Autodesk Fusion 360 part; units mm, degrees
(part 2 of 2)
  arc A38 (5.901, -3.7653) -> (6.2114, -3.2278) centre (0, 0) ccw
  spline S19 degree 5 poles (5.2406, -2.0798) (5.2443, -2.0812) (5.2517, -2.0843) (5.2626, -2.0893) (5.2768, -2.0965) (5.2942, -2.1064) (5.3113, -2.117) (5.3283, -2.128) (5.3451, -2.1393) (5.3619, -2.1506) (5.3786, -2.1622) (5.3952, -2.174) (5.4117, -2.186) (5.428, -2.1983) (5.4442, -2.211) (5.4602, -2.2239) (5.4761, -2.2372) (5.4919, -2.2506) (5.5076, -2.2642) (5.5232, -2.278) (5.5387, -2.2919) (5.5541, -2.3061) (5.5694, -2.3204) (5.5846, -2.3349) (5.5997, -2.3497) (5.6147, -2.3646) (5.6296, -2.3797) (5.6444, -2.395) (5.6591, -2.4104) (5.6737, -2.426) (5.6882, -2.4418) (5.7026, -2.4577) (5.717, -2.4738) (5.7312, -2.49) (5.7453, -2.5064) (5.7593, -2.5229) (5.7733, -2.5396) (5.7871, -2.5565) (5.8008, -2.5735) (5.8145, -2.5906) (5.828, -2.6079) (5.8415, -2.6253) (5.8549, -2.6428) (5.8681, -2.6605) (5.8813, -2.6784) (5.8944, -2.6963) (5.9074, -2.7144) (5.9203, -2.7326) (5.9331, -2.751) (5.9458, -2.7695) (5.9584, -2.7881) (5.9709, -2.8068) (5.9833, -2.8257) (5.9956, -2.8447) (6.0078, -2.8638) (6.02, -2.8831) (6.032, -2.9024) (6.0439, -2.9219) (6.0558, -2.9415) (6.0675, -2.9612) (6.0792, -2.981) (6.0907, -3.001) (6.1022, -3.0211) (6.1135, -3.0412) (6.1248, -3.0615) (6.136, -3.0819) (6.147, -3.1024) (6.158, -3.123) (6.1689, -3.1438) (6.1797, -3.1646) (6.1903, -3.1856) (6.1988, -3.2024) (6.2051, -3.2151) (6.2093, -3.2235) (6.2114, -3.2278) knots 0 0 0 0 0 0 0.01428571 0.02857143 0.04285714 0.05714286 0.07142857 0.08571429 0.1 0.11428571 0.12857143 0.14285714 0.15714286 0.17142857 0.18571429 0.2 0.21428571 0.22857143 0.24285714 0.25714286 0.27142857 0.28571429 0.3 0.31428571 0.32857143 0.34285714 0.35714286 0.37142857 0.38571429 0.4 0.41428571 0.42857143 0.44285714 0.45714286 0.47142857 0.48571429 0.5 0.51428571 0.52857143 0.54285714 0.55714286 0.57142857 0.58571429 0.6 0.61428571 0.62857143 0.64285714 0.65714286 0.67142857 0.68571429 0.7 0.71428571 0.72857143 0.74285714 0.75714286 0.77142857 0.78571429 0.8 0.81428571 0.82857143 0.84285714 0.85714286 0.87142857 0.88571429 0.9 0.91428571 0.92857143 0.94285714 0.95714286 0.97142857 0.98571429 1 1 1 1 1 1
  line L19 (5.2406, -2.0798) -> (4.8563, -1.9265)
  arc A39 (4.5613, -1.3228) -> (4.8563, -1.9265) centre (5.0415, -1.4621) ccw
  arc A40 (4.5613, -1.3228) -> (4.6116, -1.135) centre (0, 0) ccw
  arc A41 (5.1689, -0.7597) -> (4.6116, -1.135) centre (5.0971, -1.2545) ccw
  line L20 (5.1689, -0.7597) -> (5.5783, -0.8192)
  spline S20 degree 5 poles (5.5783, -0.8192) (5.5823, -0.8197) (5.5902, -0.8208) (5.6021, -0.8219) (5.6181, -0.8228) (5.6381, -0.8229) (5.6583, -0.8223) (5.6784, -0.8212) (5.6986, -0.8199) (5.7188, -0.8184) (5.7391, -0.8168) (5.7593, -0.8149) (5.7796, -0.8127) (5.7999, -0.8102) (5.8203, -0.8073) (5.8406, -0.8041) (5.861, -0.8006) (5.8814, -0.7969) (5.9018, -0.793) (5.9222, -0.7888) (5.9426, -0.7845) (5.9631, -0.7799) (5.9835, -0.7752) (6.0039, -0.7702) (6.0244, -0.765) (6.0448, -0.7596) (6.0653, -0.7539) (6.0857, -0.7481) (6.1061, -0.7421) (6.1266, -0.7359) (6.147, -0.7295) (6.1675, -0.7229) (6.1879, -0.7161) (6.2083, -0.7092) (6.2288, -0.7021) (6.2492, -0.6947) (6.2696, -0.6873) (6.29, -0.6796) (6.3104, -0.6717) (6.3308, -0.6637) (6.3512, -0.6555) (6.3715, -0.6472) (6.3919, -0.6387) (6.4122, -0.63) (6.4325, -0.6211) (6.4528, -0.6121) (6.4731, -0.6029) (6.4934, -0.5936) (6.5137, -0.5841) (6.5339, -0.5744) (6.5541, -0.5646) (6.5743, -0.5546) (6.5945, -0.5445) (6.6147, -0.5342) (6.6348, -0.5238) (6.655, -0.5132) (6.6751, -0.5024) (6.6951, -0.4915) (6.7152, -0.4805) (6.7352, -0.4693) (6.7552, -0.4579) (6.7752, -0.4464) (6.7952, -0.4348) (6.8151, -0.423) (6.835, -0.4111) (6.8549, -0.399) (6.8747, -0.3867) (6.8945, -0.3744) (6.9143, -0.3619) (6.9341, -0.3492) (6.9538, -0.3364) (6.9695, -0.3261) (6.9813, -0.3182) (6.9892, -0.313) (6.9931, -0.3103) knots 0 0 0 0 0 0 0.01428571 0.02857143 0.04285714 0.05714286 0.07142857 0.08571429 0.1 0.11428571 0.12857143 0.14285714 0.15714286 0.17142857 0.18571429 0.2 0.21428571 0.22857143 0.24285714 0.25714286 0.27142857 0.28571429 0.3 0.31428571 0.32857143 0.34285714 0.35714286 0.37142857 0.38571429 0.4 0.41428571 0.42857143 0.44285714 0.45714286 0.47142857 0.48571429 0.5 0.51428571 0.52857143 0.54285714 0.55714286 0.57142857 0.58571429 0.6 0.61428571 0.62857143 0.64285714 0.65714286 0.67142857 0.68571429 0.7 0.71428571 0.72857143 0.74285714 0.75714286 0.77142857 0.78571429 0.8 0.81428571 0.82857143 0.84285714 0.85714286 0.87142857 0.88571429 0.9 0.91428571 0.92857143 0.94285714 0.95714286 0.97142857 0.98571429 1 1 1 1 1 1
  arc A42 (6.9931, -0.3103) -> (6.9931, 0.3103) centre (0, 0) ccw
  spline S21 degree 5 poles (5.5783, 0.8192) (5.5823, 0.8197) (5.5902, 0.8208) (5.6021, 0.8219) (5.6181, 0.8228) (5.6381, 0.8229) (5.6583, 0.8223) (5.6784, 0.8212) (5.6986, 0.8199) (5.7188, 0.8184) (5.7391, 0.8168) (5.7593, 0.8149) (5.7796, 0.8127) (5.7999, 0.8102) (5.8203, 0.8073) (5.8406, 0.8041) (5.861, 0.8006) (5.8814, 0.7969) (5.9018, 0.793) (5.9222, 0.7888) (5.9426, 0.7845) (5.9631, 0.7799) (5.9835, 0.7752) (6.0039, 0.7702) (6.0244, 0.765) (6.0448, 0.7596) (6.0653, 0.7539) (6.0857, 0.7481) (6.1061, 0.7421) (6.1266, 0.7359) (6.147, 0.7295) (6.1675, 0.7229) (6.1879, 0.7161) (6.2083, 0.7092) (6.2288, 0.7021) (6.2492, 0.6947) (6.2696, 0.6873) (6.29, 0.6796) (6.3104, 0.6717) (6.3308, 0.6637) (6.3512, 0.6555) (6.3715, 0.6472) (6.3919, 0.6387) (6.4122, 0.63) (6.4325, 0.6211) (6.4528, 0.6121) (6.4731, 0.6029) (6.4934, 0.5936) (6.5137, 0.5841) (6.5339, 0.5744) (6.5541, 0.5646) (6.5743, 0.5546) (6.5945, 0.5445) (6.6147, 0.5342) (6.6348, 0.5238) (6.655, 0.5132) (6.6751, 0.5024) (6.6951, 0.4915) (6.7152, 0.4805) (6.7352, 0.4693) (6.7552, 0.4579) (6.7752, 0.4464) (6.7952, 0.4348) (6.8151, 0.423) (6.835, 0.4111) (6.8549, 0.399) (6.8747, 0.3867) (6.8945, 0.3744) (6.9143, 0.3619) (6.9341, 0.3492) (6.9538, 0.3364) (6.9695, 0.3261) (6.9813, 0.3182) (6.9892, 0.313) (6.9931, 0.3103) knots 0 0 0 0 0 0 0.01428571 0.02857143 0.04285714 0.05714286 0.07142857 0.08571429 0.1 0.11428571 0.12857143 0.14285714 0.15714286 0.17142857 0.18571429 0.2 0.21428571 0.22857143 0.24285714 0.25714286 0.27142857 0.28571429 0.3 0.31428571 0.32857143 0.34285714 0.35714286 0.37142857 0.38571429 0.4 0.41428571 0.42857143 0.44285714 0.45714286 0.47142857 0.48571429 0.5 0.51428571 0.52857143 0.54285714 0.55714286 0.57142857 0.58571429 0.6 0.61428571 0.62857143 0.64285714 0.65714286 0.67142857 0.68571429 0.7 0.71428571 0.72857143 0.74285714 0.75714286 0.77142857 0.78571429 0.8 0.81428571 0.82857143 0.84285714 0.85714286 0.87142857 0.88571429 0.9 0.91428571 0.92857143 0.94285714 0.95714286 0.97142857 0.98571429 1 1 1 1 1 1
  line L21 (5.5783, 0.8192) -> (5.1689, 0.7597)
  arc A43 (4.6116, 1.135) -> (5.1689, 0.7597) centre (5.0971, 1.2545) ccw
  arc A44 (4.6116, 1.135) -> (4.5613, 1.3228) centre (0, 0) ccw
  arc A45 (4.8563, 1.9265) -> (4.5613, 1.3228) centre (5.0415, 1.4621) ccw
  line L22 (4.8563, 1.9265) -> (5.2406, 2.0798)
  spline S22 degree 5 poles (5.2406, 2.0798) (5.2443, 2.0812) (5.2517, 2.0843) (5.2626, 2.0893) (5.2768, 2.0965) (5.2942, 2.1064) (5.3113, 2.117) (5.3283, 2.128) (5.3451, 2.1393) (5.3619, 2.1506) (5.3786, 2.1622) (5.3952, 2.174) (5.4117, 2.186) (5.428, 2.1983) (5.4442, 2.211) (5.4602, 2.2239) (5.4761, 2.2372) (5.4919, 2.2506) (5.5076, 2.2642) (5.5232, 2.278) (5.5387, 2.2919) (5.5541, 2.3061) (5.5694, 2.3204) (5.5846, 2.3349) (5.5997, 2.3497) (5.6147, 2.3646) (5.6296, 2.3797) (5.6444, 2.395) (5.6591, 2.4104) (5.6737, 2.426) (5.6882, 2.4418) (5.7026, 2.4577) (5.717, 2.4738) (5.7312, 2.49) (5.7453, 2.5064) (5.7593, 2.5229) (5.7733, 2.5396) (5.7871, 2.5565) (5.8008, 2.5735) (5.8145, 2.5906) (5.828, 2.6079) (5.8415, 2.6253) (5.8549, 2.6428) (5.8681, 2.6605) (5.8813, 2.6784) (5.8944, 2.6963) (5.9074, 2.7144) (5.9203, 2.7326) (5.9331, 2.751) (5.9458, 2.7695) (5.9584, 2.7881) (5.9709, 2.8068) (5.9833, 2.8257) (5.9956, 2.8447) (6.0078, 2.8638) (6.02, 2.8831) (6.032, 2.9024) (6.0439, 2.9219) (6.0558, 2.9415) (6.0675, 2.9612) (6.0792, 2.981) (6.0907, 3.001) (6.1022, 3.0211) (6.1135, 3.0412) (6.1248, 3.0615) (6.136, 3.0819) (6.147, 3.1024) (6.158, 3.123) (6.1689, 3.1438) (6.1797, 3.1646) (6.1903, 3.1856) (6.1988, 3.2024) (6.2051, 3.2151) (6.2093, 3.2235) (6.2114, 3.2278) knots 0 0 0 0 0 0 0.01428571 0.02857143 0.04285714 0.05714286 0.07142857 0.08571429 0.1 0.11428571 0.12857143 0.14285714 0.15714286 0.17142857 0.18571429 0.2 0.21428571 0.22857143 0.24285714 0.25714286 0.27142857 0.28571429 0.3 0.31428571 0.32857143 0.34285714 0.35714286 0.37142857 0.38571429 0.4 0.41428571 0.42857143 0.44285714 0.45714286 0.47142857 0.48571429 0.5 0.51428571 0.52857143 0.54285714 0.55714286 0.57142857 0.58571429 0.6 0.61428571 0.62857143 0.64285714 0.65714286 0.67142857 0.68571429 0.7 0.71428571 0.72857143 0.74285714 0.75714286 0.77142857 0.78571429 0.8 0.81428571 0.82857143 0.84285714 0.85714286 0.87142857 0.88571429 0.9 0.91428571 0.92857143 0.94285714 0.95714286 0.97142857 0.98571429 1 1 1 1 1 1
  arc A46 (6.2114, 3.2278) -> (5.901, 3.7653) centre (0, 0) ccw
  spline S23 degree 5 poles (4.4214, 3.4986) (4.4245, 3.5011) (4.4309, 3.5059) (4.4406, 3.5129) (4.454, 3.5216) (4.4713, 3.5317) (4.4891, 3.5412) (4.5071, 3.5504) (4.5252, 3.5594) (4.5434, 3.5682) (4.5618, 3.5769) (4.5803, 3.5854) (4.599, 3.5936) (4.6178, 3.6016) (4.6369, 3.6093) (4.6561, 3.6167) (4.6755, 3.6239) (4.695, 3.6308) (4.7146, 3.6376) (4.7344, 3.6442) (4.7542, 3.6507) (4.7742, 3.657) (4.7943, 3.6631) (4.8144, 3.669) (4.8348, 3.6747) (4.8552, 3.6802) (4.8757, 3.6856) (4.8963, 3.6907) (4.917, 3.6957) (4.9378, 3.7006) (4.9587, 3.7053) (4.9797, 3.7098) (5.0008, 3.7142) (5.022, 3.7184) (5.0432, 3.7224) (5.0646, 3.7263) (5.086, 3.73) (5.1075, 3.7335) (5.1291, 3.7369) (5.1508, 3.7402) (5.1725, 3.7433) (5.1943, 3.7462) (5.2162, 3.749) (5.2381, 3.7517) (5.2602, 3.7542) (5.2823, 3.7565) (5.3044, 3.7587) (5.3267, 3.7608) (5.349, 3.7627) (5.3713, 3.7644) (5.3937, 3.766) (5.4162, 3.7675) (5.4388, 3.7688) (5.4614, 3.77) (5.4841, 3.771) (5.5068, 3.7719) (5.5296, 3.7726) (5.5524, 3.7732) (5.5753, 3.7737) (5.5982, 3.774) (5.6212, 3.7742) (5.6443, 3.7742) (5.6674, 3.7741) (5.6906, 3.7739) (5.7138, 3.7735) (5.737, 3.773) (5.7603, 3.7723) (5.7836, 3.7715) (5.807, 3.7705) (5.8305, 3.7694) (5.8539, 3.7682) (5.8728, 3.7671) (5.8869, 3.7663) (5.8963, 3.7656) (5.901, 3.7653) knots 0 0 0 0 0 0 0.01428571 0.02857143 0.04285714 0.05714286 0.07142857 0.08571429 0.1 0.11428571 0.12857143 0.14285714 0.15714286 0.17142857 0.18571429 0.2 0.21428571 0.22857143 0.24285714 0.25714286 0.27142857 0.28571429 0.3 0.31428571 0.32857143 0.34285714 0.35714286 0.37142857 0.38571429 0.4 0.41428571 0.42857143 0.44285714 0.45714286 0.47142857 0.48571429 0.5 0.51428571 0.52857143 0.54285714 0.55714286 0.57142857 0.58571429 0.6 0.61428571 0.62857143 0.64285714 0.65714286 0.67142857 0.68571429 0.7 0.71428571 0.72857143 0.74285714 0.75714286 0.77142857 0.78571429 0.8 0.81428571 0.82857143 0.84285714 0.85714286 0.87142857 0.88571429 0.9 0.91428571 0.92857143 0.94285714 0.95714286 0.97142857 0.98571429 1 1 1 1 1 1
  line L23 (4.4214, 3.4986) -> (4.0966, 3.2424)
  arc A47 (3.4262, 3.2887) -> (4.0966, 3.2424) centre (3.7869, 3.635) ccw
  arc A48 (3.4262, 3.2887) -> (3.2887, 3.4262) centre (0, 0) ccw
  circle A49 centre (0, 0) radius 2.5
  line L24 (1.9209, -1.6) -> (-1.9209, -1.6)
  dimension "d17" = 1.6
  constraint coincident A49 L24.start
  constraint coincident A49 L24.end
  constraint horizontal L24
  measures "d17" distance of A0.centre L24
extrude "Extrusion3" add sketch "Esquisse2 (2)" against normal up to surface (4.7 mm away) contours A0 A49 L24 picked at (-0.5559, -1.6875) bodies 1 in component "Spur Gear (12 teeth)"
sketch "Esquisse1 (2)" plane through (0, 0, 0) normal (0, 0, 1) x (1, 0, 0) in component "Spur Gear (42 teeth)"
  circle A0 centre (0, 0) radius 19.7492
  circle A1 centre (0, 0) radius 15
extrude "Extrusion1'" add sketch "Esquisse1 (2)" along normal blind 4.7 separate body makes body 2 in component "Spur Gear (42 teeth)"
sketch "Esquisse2 (3)" plane through (0, 0, 0) normal (0, 0, 1) x (1, 0, 0) in component "Spur Gear (42 teeth)"
  spline S0 degree 5 poles (19.7066, -1.0317) (19.7131, -1.0317) (19.7263, -1.0318) (19.746, -1.0317) (19.7723, -1.0312) (19.8053, -1.0301) (19.8382, -1.0284) (19.8711, -1.0262) (19.9041, -1.0236) (19.937, -1.0204) (19.97, -1.0169) (20.003, -1.013) (20.036, -1.0087) (20.0689, -1.0042) (20.1019, -0.9994) (20.1349, -0.9944) (20.1678, -0.9891) (20.2008, -0.9835) (20.2337, -0.9776) (20.2667, -0.9715) (20.2996, -0.9652) (20.3326, -0.9586) (20.3655, -0.9517) (20.3984, -0.9447) (20.4314, -0.9374) (20.4643, -0.93) (20.4972, -0.9223) (20.5301, -0.9144) (20.563, -0.9063) (20.5958, -0.898) (20.6287, -0.8895) (20.6616, -0.8808) (20.6944, -0.872) (20.7273, -0.8629) (20.7601, -0.8536) (20.7929, -0.8442) (20.8257, -0.8346) (20.8585, -0.8248) (20.8913, -0.8148) (20.9241, -0.8047) (20.9568, -0.7944) (20.9896, -0.7839) (21.0223, -0.7732) (21.055, -0.7624) (21.0877, -0.7514) (21.1204, -0.7403) (21.1531, -0.729) (21.1857, -0.7175) (21.2184, -0.7059) (21.251, -0.6941) (21.2836, -0.6821) (21.3162, -0.67) (21.3488, -0.6578) (21.3814, -0.6454) (21.4139, -0.6328) (21.4465, -0.6201) (21.479, -0.6072) (21.5115, -0.5942) (21.544, -0.5811) (21.5764, -0.5678) (21.6089, -0.5544) (21.6413, -0.5408) (21.6737, -0.527) (21.7061, -0.5132) (21.7385, -0.4992) (21.7708, -0.485) (21.8031, -0.4707) (21.8354, -0.4563) (21.8677, -0.4417) (21.9, -0.427) (21.9323, -0.4122) (21.958, -0.4002) (21.9774, -0.3911) (21.9902, -0.3851) (21.9967, -0.382) knots 0 0 0 0 0 0 0.01428571 0.02857143 0.04285714 0.05714286 0.07142857 0.08571429 0.1 0.11428571 0.12857143 0.14285714 0.15714286 0.17142857 0.18571429 0.2 0.21428571 0.22857143 0.24285714 0.25714286 0.27142857 0.28571429 0.3 0.31428571 0.32857143 0.34285714 0.35714286 0.37142857 0.38571429 0.4 0.41428571 0.42857143 0.44285714 0.45714286 0.47142857 0.48571429 0.5 0.51428571 0.52857143 0.54285714 0.55714286 0.57142857 0.58571429 0.6 0.61428571 0.62857143 0.64285714 0.65714286 0.67142857 0.68571429 0.7 0.71428571 0.72857143 0.74285714 0.75714286 0.77142857 0.78571429 0.8 0.81428571 0.82857143 0.84285714 0.85714286 0.87142857 0.88571429 0.9 0.91428571 0.92857143 0.94285714 0.95714286 0.97142857 0.98571429 1 1 1 1 1 1
  spline S1 degree 5 poles (19.7066, 1.0317) (19.7131, 1.0317) (19.7263, 1.0318) (19.746, 1.0317) (19.7723, 1.0312) (19.8053, 1.0301) (19.8382, 1.0284) (19.8711, 1.0262) (19.9041, 1.0236) (19.937, 1.0204) (19.97, 1.0169) (20.003, 1.013) (20.036, 1.0087) (20.0689, 1.0042) (20.1019, 0.9994) (20.1349, 0.9944) (20.1678, 0.9891) (20.2008, 0.9835) (20.2337, 0.9776) (20.2667, 0.9715) (20.2996, 0.9652) (20.3326, 0.9586) (20.3655, 0.9517) (20.3984, 0.9447) (20.4314, 0.9374) (20.4643, 0.93) (20.4972, 0.9223) (20.5301, 0.9144) (20.563, 0.9063) (20.5958, 0.898) (20.6287, 0.8895) (20.6616, 0.8808) (20.6944, 0.872) (20.7273, 0.8629) (20.7601, 0.8536) (20.7929, 0.8442) (20.8257, 0.8346) (20.8585, 0.8248) (20.8913, 0.8148) (20.9241, 0.8047) (20.9568, 0.7944) (20.9896, 0.7839) (21.0223, 0.7732) (21.055, 0.7624) (21.0877, 0.7514) (21.1204, 0.7403) (21.1531, 0.729) (21.1857, 0.7175) (21.2184, 0.7059) (21.251, 0.6941) (21.2836, 0.6821) (21.3162, 0.67) (21.3488, 0.6578) (21.3814, 0.6454) (21.4139, 0.6328) (21.4465, 0.6201) (21.479, 0.6072) (21.5115, 0.5942) (21.544, 0.5811) (21.5764, 0.5678) (21.6089, 0.5544) (21.6413, 0.5408) (21.6737, 0.527) (21.7061, 0.5132) (21.7385, 0.4992) (21.7708, 0.485) (21.8031, 0.4707) (21.8354, 0.4563) (21.8677, 0.4417) (21.9, 0.427) (21.9323, 0.4122) (21.958, 0.4002) (21.9774, 0.3911) (21.9902, 0.3851) (21.9967, 0.382) knots 0 0 0 0 0 0 0.01428571 0.02857143 0.04285714 0.05714286 0.07142857 0.08571429 0.1 0.11428571 0.12857143 0.14285714 0.15714286 0.17142857 0.18571429 0.2 0.21428571 0.22857143 0.24285714 0.25714286 0.27142857 0.28571429 0.3 0.31428571 0.32857143 0.34285714 0.35714286 0.37142857 0.38571429 0.4 0.41428571 0.42857143 0.44285714 0.45714286 0.47142857 0.48571429 0.5 0.51428571 0.52857143 0.54285714 0.55714286 0.57142857 0.58571429 0.6 0.61428571 0.62857143 0.64285714 0.65714286 0.67142857 0.68571429 0.7 0.71428571 0.72857143 0.74285714 0.75714286 0.77142857 0.78571429 0.8 0.81428571 0.82857143 0.84285714 0.85714286 0.87142857 0.88571429 0.9 0.91428571 0.92857143 0.94285714 0.95714286 0.97142857 0.98571429 1 1 1 1 1 1
  arc A0 (21.9967, -0.382) -> (21.9967, 0.382) centre (0, 0) ccw
  line L0 (19.7066, 1.0317) -> (19.7066, -1.0317)
  point P0 (19.8689, -1.0263)
  point P1 (20.0319, -1.0092)
  point P2 (20.1952, -0.9844)
  point P3 (20.3588, -0.9531)
  point P4 (20.5226, -0.9162)
  point P5 (20.6864, -0.8741)
  point P6 (20.8504, -0.8272)
  point P7 (21.0143, -0.7758)
  point P8 (21.1783, -0.7201)
  point P9 (21.3422, -0.6602)
  point P10 (21.5061, -0.5964)
  point P11 (21.6698, -0.5287)
  point P12 (21.8333, -0.4572)
  point P13 (19.8689, 1.0263)
  point P14 (20.0319, 1.0092)
  point P15 (20.1952, 0.9844)
  point P16 (20.3588, 0.9531)
  point P17 (20.5226, 0.9162)
  point P18 (20.6864, 0.8741)
  point P19 (20.8504, 0.8272)
  point P20 (21.0143, 0.7758)
  point P21 (21.1783, 0.7201)
  point P22 (21.3422, 0.6602)
  point P23 (21.5061, 0.5964)
  point P24 (21.6698, 0.5287)
  point P25 (21.8333, 0.4572)
extrude "Extrusion2'" add sketch "Esquisse2 (3)" along normal blind 4.7 bodies 2 in component "Spur Gear (42 teeth)"
fillet "Congé1'" radius 0.5 2 edges at (19.7222, 1.0317, 2.35) (19.7222, -1.0317, 2.35) on bodies 2 in component "Spur Gear (42 teeth)"
pattern_circular "Réseau C1'" count 42 over 360 about axis through (0, 0, 0) along (0, 0, 1) of "Extrusion2'", "Congé1'" in component "Spur Gear (42 teeth)"
sketch "Esquisse3 (2)" plane through (0, 0, 0) normal (0, 0, 1) x (1, 0, 0) in component "Spur Gear (42 teeth)"
  circle A0 centre (0, 0) radius 21 construction
component "Spur Gear (12 teeth)" placed x (1, 0, 0) y (0, 1, 0) z (0, 0, 1) at (0, 0, 0)
component "Spur Gear (42 teeth)" placed x (1, 0, 0) y (0, 1, 0) z (0, 0, 1) at (0, 0, 0)

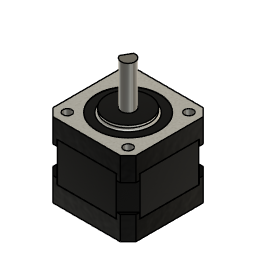
design "Nema-17"
Autodesk Fusion 360 part; units mm, degrees
sketch "Esquisse1" plane through (0, 0, 0) normal (0, 0, 1) x (1, 0, 0)
  line L0 (21.15, 21.15) -> (-21.15, 21.15)
  line L1 (-21.15, 21.15) -> (-21.15, -21.15)
  line L2 (-21.15, -21.15) -> (21.15, -21.15)
  line L3 (21.15, -21.15) -> (21.15, 21.15)
  line L4 (21.15, 21.15) -> (-21.15, -21.15) construction
  line L5 (-21.15, 21.15) -> (21.15, -21.15) construction
  circle A0 centre (0, 0) radius 2.5
  circle A1 centre (-15.5, 15.5) radius 2.25
  line L6 (-21.15, 0) -> (21.15, 0) construction
  line L7 (0, 21.15) -> (0, -21.15) construction
  circle A2 centre (15.5, 15.5) radius 2.25
  circle A3 centre (-15.5, -15.5) radius 2.25
  circle A4 centre (15.5, -15.5) radius 2.25
  line L8 (-15.15, 21.15) -> (-21.15, 15.15)
  line L9 (15.15, 21.15) -> (21.15, 15.15)
  line L10 (-15.15, -21.15) -> (-21.15, -15.15)
  line L11 (15.15, -21.15) -> (21.15, -15.15)
  dimension "d1" = 42.3
  dimension "d2" = 42.3
  dimension "d3" = 5
  dimension "d4" = 4.5
  dimension "d7" = 15.5
  dimension "d8" = 15.5
  dimension "d11" = 6
  constraint horizontal L0
  constraint perpendicular L0 L1
  constraint parallel L0 L2
  constraint parallel L1 L3
  constraint coincident L4 A0.centre
  constraint coincident L5 A0.centre
  constraint coincident A0.centre origin
  constraint midpoint L1 L6.start
  constraint midpoint L3 L6.end
  constraint midpoint L0 L7.start
  constraint midpoint L2 L7.end
  constraint symmetric A1 L7 A2
  constraint symmetric A1 L6 A3
  constraint symmetric L6 A2 A4
  constraint coincident L0 L8.start
  constraint coincident L1 L8.end
  constraint perpendicular L5 L8
  constraint symmetric L7 L8.start L9.start
  constraint symmetric L7 L8.end L9.end
  constraint symmetric L6 L8.start L10.start
  constraint symmetric L6 L8.end L10.end
  constraint symmetric L6 L9.start L11.start
  constraint symmetric L6 L9.end L11.end
  measures "d1" distance of L1.end L2.end
  measures "d2" distance of L0.end L1.end
  measures "d3" diameter of A0
  measures "d4" diameter of A1
  measures "d7" distance of A1.centre L6
  measures "d8" distance of A1.centre L7
  measures "d11" distance of L0.end L8.start
extrude "Extrusion1" add sketch "Esquisse1" against normal blind 9 makes body 1
extrude "Extrusion2" add sketch "Esquisse1" along normal blind 3 contours L0 L3 L9 | L0 L1 L8 | L2 L3 L11 | L1 L2 L10 bodies 1
chamfer "Chanfrein1" distance 4 angle 45 4 edges at (-21.15, 21.15, -3) (21.15, 21.15, -3) (21.15, -21.15, -3) (-21.15, -21.15, -3) on bodies 1
sketch "Esquisse2" plane through (0, 0, 0) normal (0, 0, 1) x (-1, 0, 0)
  line L0 (15.15, -21.15) -> (21.15, -15.15)
  line L1 (21.15, -15.15) -> (21.15, 15.15)
  line L2 (21.15, 15.15) -> (15.15, 21.15)
  line L3 (15.15, 21.15) -> (-15.15, 21.15)
  line L4 (-15.15, 21.15) -> (-21.15, 15.15)
  line L5 (-21.15, 15.15) -> (-21.15, -15.15)
  line L6 (-21.15, -15.15) -> (-15.15, -21.15)
  line L7 (-15.15, -21.15) -> (15.15, -21.15)
  circle A0 centre (-15.5, -15.5) radius 2.25
  circle A1 centre (0, 0) radius 2.5
  circle A2 centre (-15.5, 15.5) radius 2.25
  circle A3 centre (15.5, 15.5) radius 2.25
  circle A4 centre (15.5, -15.5) radius 2.25
  line L8 (20.95, -15.0672) -> (20.95, 15.0672)
  line L9 (20.95, 15.0672) -> (15.0672, 20.95)
  line L10 (15.0672, 20.95) -> (-15.0672, 20.95)
  line L11 (-15.0672, 20.95) -> (-20.95, 15.0672)
  line L12 (-20.95, 15.0672) -> (-20.95, -15.0672)
  line L13 (-20.95, -15.0672) -> (-15.0672, -20.95)
  line L14 (-15.0672, -20.95) -> (15.0672, -20.95)
  line L15 (15.0672, -20.95) -> (20.95, -15.0672)
  line L16 (20.95, -15.0672) -> (21.15, -14.8672)
  line L17 (15.0672, -20.95) -> (14.8672, -21.15)
  line L18 (-15.0672, -20.95) -> (-14.8672, -21.15)
  line L19 (-20.95, -15.0672) -> (-21.15, -14.8672)
  line L20 (-20.95, 15.0672) -> (-21.15, 14.8672)
  line L21 (-15.0672, 20.95) -> (-14.8672, 21.15)
  line L22 (15.0672, 20.95) -> (14.8672, 21.15)
  line L23 (20.95, 15.0672) -> (21.15, 14.8672)
  line L24 (-14.9672, -21.05) -> (14.9672, -21.05)
  line L25 (21.05, -14.9672) -> (21.05, 14.9672)
  line L26 (14.9672, 21.05) -> (-14.9672, 21.05)
  line L27 (-21.05, 14.9672) -> (-21.05, -14.9672)
  dimension "d15" = -0.2
  constraint parallel L15 L16
  constraint coincident L7 L17.end
  constraint parallel L15 L17
  constraint coincident L7 L18.end
  constraint perpendicular L17 L18
  constraint coincident L5 L19.end
  constraint parallel L13 L19
  constraint coincident L5 L20.end
  constraint perpendicular L19 L20
  constraint coincident L3 L21.end
  constraint parallel L11 L21
  constraint coincident L3 L22.end
  constraint parallel L9 L22
  constraint coincident L1 L23.end
  constraint parallel L9 L23
  constraint midpoint L18 L24.start
  constraint midpoint L17 L24.end
  constraint midpoint L16 L25.start
  constraint midpoint L23 L25.end
  constraint parallel L8 L25
  constraint midpoint L22 L26.start
  constraint midpoint L21 L26.end
  constraint midpoint L20 L27.start
  constraint midpoint L19 L27.end
extrude "Extrusion3" add sketch "Esquisse2" along normal blind 17 contours L14 L17 L18 L24 | L8 L16 L23 L25 | L8 L9 L10 L11 L12 L13 L14 L15 | L12 L19 L20 L27 | L10 L21 L22 L26 bodies 1
sketch "Esquisse3" plane through (0, 0, 17) normal (0, 0, 1) x (-1, 0, 0)
  circle A0 centre (0, 0) radius 2.5
  line L0 (-14.9672, 21.05) -> (-21.05, 14.9672)
  line L1 (-21.05, 14.9672) -> (-21.05, -14.9672)
  line L2 (-21.05, -14.9672) -> (-14.9672, -21.05)
  line L3 (-14.9672, -21.05) -> (14.9672, -21.05)
  line L4 (14.9672, -21.05) -> (21.05, -14.9672)
  line L5 (21.05, -14.9672) -> (21.05, 14.9672)
  line L6 (21.05, 14.9672) -> (14.9672, 21.05)
  line L7 (14.9672, 21.05) -> (-14.9672, 21.05)
  line L8 (21.15, 17.15) -> (17.15, 21.15)
  line L9 (17.15, 21.15) -> (15.15, 21.15)
  line L10 (15.15, 21.15) -> (21.15, 15.15)
  line L11 (21.15, 15.15) -> (21.15, 17.15)
  line L12 (17.15, -21.15) -> (21.15, -17.15)
  line L13 (21.15, -17.15) -> (21.15, -15.15)
  line L14 (21.15, -15.15) -> (15.15, -21.15)
  line L15 (15.15, -21.15) -> (17.15, -21.15)
  line L16 (-21.15, -17.15) -> (-17.15, -21.15)
  line L17 (-17.15, -21.15) -> (-15.15, -21.15)
  line L18 (-15.15, -21.15) -> (-21.15, -15.15)
  line L19 (-21.15, -15.15) -> (-21.15, -17.15)
  line L20 (-17.15, 21.15) -> (-21.15, 17.15)
  line L21 (-21.15, 17.15) -> (-21.15, 15.15)
  line L22 (-21.15, 15.15) -> (-15.15, 21.15)
  line L23 (-15.15, 21.15) -> (-17.15, 21.15)
  line L24 (17.15, 21.15) -> (21.15, 17.15)
  line L25 (21.15, 17.15) -> (21.15, -17.15)
  line L26 (21.15, -17.15) -> (17.15, -21.15)
  line L27 (17.15, -21.15) -> (-17.15, -21.15)
  line L28 (-17.15, -21.15) -> (-21.15, -17.15)
  line L29 (-21.15, -17.15) -> (-21.15, 17.15)
  line L30 (-21.15, 17.15) -> (-17.15, 21.15)
  line L31 (-17.15, 21.15) -> (17.15, 21.15)
  circle A1 centre (-15.5, -15.5) radius 2.25
  circle A2 centre (0, 0) radius 2.5
  circle A3 centre (-15.5, 15.5) radius 2.25
  circle A4 centre (15.5, 15.5) radius 2.25
  circle A5 centre (15.5, -15.5) radius 2.25
  circle A6 centre (15.5, 15.5) radius 2.25
  circle A7 centre (-15.5, -15.5) radius 2.25
  circle A8 centre (15.5, -15.5) radius 2.25
  circle A9 centre (-15.5, 15.5) radius 2.25
extrude "Extrusion4" add sketch "Esquisse3" along normal blind 3 contours L0 L1 L2 L3 L4 L5 L6 L7 | L8 L9 L10 L11 L24 L25 L31 | L12 L13 L14 L15 L25 L26 L27 | L20 L21 L22 L23 L29 L30 L31 | L16 L17 L18 L19 L27 L28 L29 bodies 1 makes body 2 at (-19.15, 17.15, 18) makes body 3 at (-17.15, -19.15, 18) makes body 4 at (17.15, 19.15, 18) makes body 5 at (19.15, -17.15, 18)
sketch "Esquisse4" plane through (0, 0, 20) normal (0, 0, 1) x (-1, 0, 0)
  circle A0 centre (-15.5, -15.5) radius 2.25
  circle A1 centre (0, 0) radius 2.5
  line L0 (14.9672, 21.05) -> (-14.9672, 21.05)
  line L1 (-14.9672, 21.05) -> (-21.05, 14.9672)
  line L2 (-21.05, 14.9672) -> (-21.05, -14.9672)
  line L3 (-21.05, -14.9672) -> (-14.9672, -21.05)
  line L4 (-14.9672, -21.05) -> (14.9672, -21.05)
  line L5 (14.9672, -21.05) -> (21.05, -14.9672)
  line L6 (21.05, -14.9672) -> (21.05, 14.9672)
  line L7 (21.05, 14.9672) -> (14.9672, 21.05)
  line L8 (-15.15, -21.15) -> (15.15, -21.15)
  line L9 (-21.15, 15.15) -> (-21.15, -15.15)
  line L10 (15.15, 21.15) -> (-15.15, 21.15)
  line L11 (21.15, -15.15) -> (21.15, 15.15)
  line L12 (17.15, 21.15) -> (15.15, 21.15)
  line L13 (15.15, 21.15) -> (21.15, 15.15)
  line L14 (21.15, 15.15) -> (21.15, 17.15)
  line L15 (21.15, 17.15) -> (17.15, 21.15)
  line L16 (-21.15, 15.15) -> (-15.15, 21.15)
  line L17 (-15.15, 21.15) -> (-17.15, 21.15)
  line L18 (-17.15, 21.15) -> (-21.15, 17.15)
  line L19 (-21.15, 17.15) -> (-21.15, 15.15)
  line L20 (-15.15, -21.15) -> (-21.15, -15.15)
  line L21 (-21.15, -15.15) -> (-21.15, -17.15)
  line L22 (-21.15, -17.15) -> (-17.15, -21.15)
  line L23 (-17.15, -21.15) -> (-15.15, -21.15)
  line L24 (21.15, -15.15) -> (15.15, -21.15)
  line L25 (15.15, -21.15) -> (17.15, -21.15)
  line L26 (17.15, -21.15) -> (21.15, -17.15)
  line L27 (21.15, -17.15) -> (21.15, -15.15)
  circle A2 centre (15.5, -15.5) radius 2.25
  circle A3 centre (-15.5, 15.5) radius 2.25
  circle A4 centre (15.5, 15.5) radius 2.25
extrude "Extrusion5" add sketch "Esquisse4" along normal blind 9 contours L0 L1 L2 L3 L4 L5 L6 L7 | L8 L9 L10 L11 L13 L16 L20 L24 | L20 L21 L22 L23 | L24 L25 L26 L27 | L16 L17 L18 L19 | L12 L13 L14 L15 bodies 1 2 3 4 5
sketch "Esquisse5" plane through (0, 0, 29) normal (0, 0, 1) x (-1, 0, 0)
  circle A0 centre (0, 0) radius 2.5
  circle A1 centre (-15.5, 15.5) radius 2.25
  circle A2 centre (15.5, -15.5) radius 2.25
  circle A3 centre (-15.5, -15.5) radius 2.25
  circle A4 centre (15.5, 15.5) radius 2.25
  line L0 (21.15, -17.15) -> (21.15, 17.15)
  line L1 (21.15, 17.15) -> (17.15, 21.15)
  line L2 (17.15, 21.15) -> (-17.15, 21.15)
  line L3 (-17.15, 21.15) -> (-21.15, 17.15)
  line L4 (-21.15, 17.15) -> (-21.15, -17.15)
  line L5 (-21.15, -17.15) -> (-17.15, -21.15)
  line L6 (-17.15, -21.15) -> (17.15, -21.15)
  line L7 (17.15, -21.15) -> (21.15, -17.15)
  circle A5 centre (0, 0) radius 2.5
  circle A6 centre (0, 0) radius 16
  circle A7 centre (0, 0) radius 11
  circle A8 centre (0, 0) radius 3.5
  line L8 (2, -2.8723) -> (2, 2.8723)
  dimension "d22" = 32
  dimension "d23" = 22
  dimension "d24" = 7
  dimension "d60" = 2
  constraint concentric A5 A6
  constraint concentric A5 A7
  constraint concentric A7 A8
  constraint coincident A8 L8.start
  constraint coincident A8 L8.end
  constraint vertical L8
  measures "d22" diameter of A6
  measures "d23" diameter of A7
  measures "d24" diameter of A8
  measures "d60" distance of A0.centre L8
extrude "Extrusion6" cut sketch "Esquisse5" against normal up to surface (38 mm away) contours A0 A5 A8 L8 | A0 A5 A8 L8 bodies 1
extrude "Extrusion7" cut sketch "Esquisse5" against normal blind 0.2 contours A6 bodies 1
extrude "Extrusion8" add sketch "Esquisse5" along normal blind 2 contours A7 bodies 1
extrude "Extrusion9" add sketch "Esquisse5" along normal blind 24 and the other way blind 38 separate body contours A0 A5 L8 | A0 A5 A8 L8 | A0 A5 L8 | A0 A5 A8 L8 makes body 6
fillet "Congé1" radius 1 1 edges at (10.2556, 3.9778, 28.8) on bodies 1
sketch "Esquisse6" plane through (-21.15, 0, 0) normal (-1, 0, 0) x (0, -1, 0)
  line L0 (17.15, -9) -> (17.15, 3)
  line L1 (17.15, 3) -> (15.15, 3)
  line L2 (15.15, 3) -> (15.15, 0)
  line L3 (15.15, 0) -> (-15.15, 0)
  line L4 (-15.15, 0) -> (-15.15, 3)
  line L5 (-15.15, 3) -> (-17.15, 3)
  line L6 (-17.15, 3) -> (-17.15, -9)
  line L7 (-17.15, -9) -> (17.15, -9)
  line L8 (5, -7) -> (-5, -7)
  line L9 (-5, -7) -> (-5, -2)
  line L10 (-5, -2) -> (5, -2)
  line L11 (5, -2) -> (5, -7)
  line L12 (5, -7) -> (-5, -2) construction
  line L13 (-5, -7) -> (5, -2) construction
  line L14 (7.5, -1.5) -> (-7.5, -1.5)
  line L15 (-7.5, -1.5) -> (-7.5, -7.5)
  line L16 (-7.5, -7.5) -> (7.5, -7.5)
  line L17 (7.5, -7.5) -> (7.5, -1.5)
  line L18 (7.5, -1.5) -> (-7.5, -7.5) construction
  line L19 (-7.5, -1.5) -> (7.5, -7.5) construction
  line L20 (-7.5, -4.5) -> (7.5, -4.5) construction
  line L21 (0, -2) -> (0, -7) construction
  circle A0 centre (-3.75, -4.5) radius 0.75
  line L22 (-2.5, -7) -> (-2.5, -2) construction
  circle A1 centre (-1.25, -4.5) radius 0.75
  circle A2 centre (1.25, -4.5) radius 0.75
  circle A3 centre (3.75, -4.5) radius 0.75
  point P0 (0, -4.5)
  point P1 (0, -4.5)
  point P2 (0, -4.5)
  point P3 (0, -4.5)
  dimension "d37" = 10
  dimension "d38" = 5
  dimension "d39" = 2
  dimension "d40" = 5
  dimension "d41" = 6
  dimension "d42" = 15
  dimension "d51" = 0.5
  dimension "d52" = 2.5
  dimension "d57" = 1.25
  dimension "d58" = 1.5
  dimension "d59" = 1.25
  constraint horizontal L8
  constraint perpendicular L8 L9
  constraint parallel L8 L10
  constraint parallel L9 L11
  constraint horizontal L14
  constraint perpendicular L14 L15
  constraint parallel L14 L16
  constraint parallel L15 L17
  constraint coincident P3 P2
  constraint midpoint L15 L20.start
  constraint midpoint L17 L20.end
  constraint coincident L19 P3
  constraint coincident L12 P3
  constraint coincident P3 L18
  constraint midpoint L10 L21.start
  constraint midpoint L8 L21.end
  constraint coincident L20 A0.centre
  constraint coincident L8 L22.start
  constraint coincident L10 L22.end
  constraint perpendicular L10 L22
  constraint symmetric A0 L22 A1
  constraint symmetric L21 A0 A3
  constraint symmetric L21 A1 A2
  measures "d37" distance of L9.end L10.end
  measures "d38" distance of L8.end L9.end
  measures "d39" distance of origin L10
  measures "d40" distance of origin L11
  measures "d41" distance of L14.end L15.end
  measures "d42" distance of L14.start L14.end
  measures "d51" distance of L10 L14
  measures "d52" distance of L9 L15
  measures "d57" distance of L9 A0.centre
  measures "d58" diameter of A0
  measures "d59" distance of A0.centre L22
extrude "Extrusion10" add sketch "Esquisse6" along normal blind 0.1 contours L8 L9 L10 L11 bodies 1 6
extrude "Extrusion12" cut sketch "Esquisse6" along normal blind 0.5 and the other way blind 5 contours A0 | A1 | A2 | A3 bodies 6 1
sketch "Esquisse7" plane through (0, 0, 53) normal (0, 0, 1) x (-1, 0, 0)
  circle A0 centre (0, 0) radius 3.5
  line L0 (2.2119, -2.7125) -> (2.2119, 2.7125)
  circle A1 centre (0, 0) radius 3.5
  line L1 (0, 0) -> (4.5, 0) construction
  circle A2 centre (0, 0) radius 3.5
  dimension "d66" = 5.425
  constraint coincident A0 L0.start
  constraint coincident A0 L0.end
  constraint coincident L0.start A1
  constraint coincident A0.centre A1.centre
  constraint horizontal L1
  constraint perpendicular L0 L1
  measures "d66" distance of L0.start L0.end
extrude "Extrusion15" cut sketch "Esquisse7" against normal blind 18 contours A0 L0 A1 A2 picked at (2.8409, -0.3398) bodies 6 1
copy_body "Corps->Comp1" bodies 6 removing the originals makes body 7 in component "Component"
component "Component" placed x (1, 0, 0) y (0, 1, 0) z (0, 0, 1) at (0, 0, 0)
named bodies: "Nema 17"
